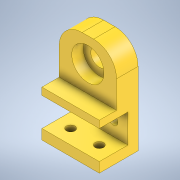
# Autodesk Inventor part: Giu truc X
Saved by Autodesk Inventor 2020 (Build 240168000, 168)
## iProperties
Created: 2021-06-03
Part Number: Giu truc X
Material: Generic
Document SubType Name: Modeling
Designer: admin
Density: 1 g/cm^3
Appearance: Glossy - Gold
Author: admin
Autodesk Inventor part; units mm, degrees
ref_plane "YZ Plane" through (0, 0, 0) normal (1, 0, 0) x (0, 1, 0)
ref_plane "XZ Plane" through (0, 0, 0) normal (0, 1, 0) x (-1, 0, 0)
ref_plane "XY Plane" through (0, 0, 0) normal (0, 0, 1) x (1, 0, 0)
sketch "Sketch1" plane through (0, 0, 0) normal (0, 0, 1) x (1, 0, 0)
  line L0 (-20, -30) -> (20, -30)
  line L1 (20, -30) -> (20, 30)
  line L2 (20, 30) -> (-20, 30)
  line L3 (-20, 30) -> (-20, -30)
  line L4 (-20, -30) -> (20, 30) construction
  line L5 (20, -30) -> (-20, 30) construction
  point P0 (0, 0)
  dimension "d0" = 40
  dimension "d1" = 60
  constraints: 12 end point, 2 midpoint, 2 parallel, 1 horizontal, 1 perpendicular
  measures "d0" distance of L2.end L1.end
  measures "d1" distance of L1.end L0.end
extrude "Extrusion1" add sketch "Sketch1" along normal blind 15
sketch "Sketch2" plane through (0, 0, 15) normal (0, 0, 1) x (1, 0, 0)
  circle A0 centre (0, 13) radius 11.25
  line L0 (-20, -30) -> (20, -30) projected
  point P0 (0, 0)
  dimension "d4" = 22.5
  dimension "d5" = 43
  constraints: 1 centre point
  measures "d4" diameter of A0
  measures "d5" distance from line of L0 A0.centre
extrude "Extrusion2" cut sketch "Sketch2" against normal blind 8
sketch "Sketch3" plane through (0, 13, 7) normal (0, 0, 1) x (1, 0, 0)
  circle A0 centre (0, 0) radius 6
  point P0 (0, -13)
  dimension "d8" = 12
  constraints: 1 centre point
  measures "d8" diameter of A0
extrude "Extrusion3" cut sketch "Sketch3" against normal through all
fillet "Fillet1" radius 16 2 edges at (20, 30, 7.5) (-20, 30, 7.5)
sketch "Sketch4" plane through (0, 0, 15) normal (0, 0, 1) x (1, 0, 0)
  line L0 (-20, 14) -> (-20, -30) projected
  line L1 (20, -30) -> (20, 14) projected
  line L2 (-20, -30) -> (20, -30)
  line L3 (20, -30) -> (20, -10)
  line L4 (20, -10) -> (-20, -10)
  line L5 (-20, -10) -> (-20, -30)
  point P0 (0, 0)
  dimension "d12" = 20
  constraints: 8 end point, 2 parallel, 1 horizontal, 1 perpendicular, 1 point on line
  measures "d12" distance of L3.end L2.end
extrude "Extrusion4" cut sketch "Sketch4" against normal blind 8
sketch "Sketch5" plane through (-20, -30, 0) normal (0, -1, 0) x (1, 0, 0)
  line L0 (0, 0) -> (40, 0) projected
  line L1 (40, 0) -> (0, 0)
  line L2 (0, 0) -> (0, 27)
  line L3 (0, 27) -> (40, 27)
  line L4 (40, 27) -> (40, 0)
  point P0 (20, 0)
  dimension "d15" = 27
  constraints: 8 end point, 2 parallel, 1 horizontal, 1 perpendicular
  measures "d15" distance of L1.end L2.end
extrude "Extrusion5" add sketch "Sketch5" along normal blind 7
sketch "Sketch6" plane through (0, 0, 7) normal (0, 0, 1) x (1, 0, 0)
  circle A0 centre (-10, -20) radius 3
  circle A1 centre (10, -20) radius 3
  line L0 (20, -30) -> (-20, -30) projected
  line L1 (0, -42) -> (0, 42) projected
  point P0 (0, 0)
  dimension "d19" = 6
  dimension "d20" = 6
  dimension "d21" = 10
  dimension "d22" = 20
  dimension "d23" = 10
  dimension "d24" = 10
  constraints: 2 centre point
  measures "d19" diameter of A0
  measures "d20" diameter of A1
  measures "d21" distance from line of L0 A0.centre
  measures "d22" distance of A1.centre A0.centre
  measures "d23" distance from line of A0.centre L1
  measures "d24" distance from line of L0 A1.centre
extrude "Extrusion6" cut sketch "Sketch6" against normal blind 7
sketch "Sketch7" plane through (-20, -37, 0) normal (0, -1, 0) x (1, 0, 0)
  circle A0 centre (30, 17) radius 3
  circle A1 centre (10, 17) radius 3
  line L0 (40, 27) -> (0, 27) projected
  point P0 (20, 0)
  dimension "d27" = 6
  dimension "d28" = 6
  dimension "d29" = 10
  dimension "d30" = 10
  dimension "d31" = 20
  dimension "d32" = 10
  constraints: 2 centre point
  measures "d27" diameter of A0
  measures "d28" diameter of A1
  measures "d29" distance from line of L0 A0.centre
  measures "d30" distance from line of L0 A1.centre
  measures "d31" distance of A1.centre A0.centre
  measures "d32" horizontal distance of point (20, 0) A0.centre
extrude "Extrusion7" cut sketch "Sketch7" against normal blind 7
sketch "Sketch8" plane through (0, 0, 15) normal (0, 0, 1) x (1, 0, 0)
  line L0 (-20, -10) -> (20, -10) projected
  line L1 (20, -10) -> (20, 14) projected
  line L2 (-20, -10) -> (20, -10)
  line L3 (20, -10) -> (20, -5)
  line L4 (20, -5) -> (-20, -5)
  line L5 (-20, -5) -> (-20, -10)
  point P0 (0, 0)
  dimension "d35" = 5
  constraints: 8 end point, 2 parallel, 1 horizontal, 1 perpendicular, 1 point on line
  measures "d35" distance of L3.end L2.end
extrude "Extrusion8" add sketch "Sketch8" along normal blind 12
body "Solid1"
